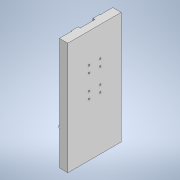
# Autodesk Inventor part: Zplita
Saved by Autodesk Inventor 2020.1 (Build 241239000, 239)
## iProperties
Created: 2023-01-09
Part Number: Zplita
Material: Типовые
Document SubType Name: Modeling
Designer: KirikDK
Density: 1 g/cm^3
Appearance: По умолчанию
Author: KirikDK
Autodesk Inventor part; units mm, degrees
ref_plane "YZ Plane" through (0, 0, 0) normal (1, 0, 0) x (0, 1, 0)
ref_plane "XZ Plane" through (0, 0, 0) normal (0, 1, 0) x (-1, 0, 0)
ref_plane "XY Plane" through (0, 0, 0) normal (0, 0, 1) x (1, 0, 0)
sketch "Эскиз1" plane through (0, 0, 0) normal (0, 1, 0) x (-1, 0, 0)
  line L0 (0, 94.5239) -> (-30, 94.5239)
  line L1 (-30, 94.5239) -> (-30, -95.4761)
  line L2 (-30, -95.4761) -> (0, -95.4761)
  line L3 (0, -95.4761) -> (0, 94.5239)
  line L4 (-30, 50.5239) -> (2, 50.5239)
  line L5 (2, 50.5239) -> (2, -51.4761)
  line L6 (2, -51.4761) -> (-30, -51.4761)
  line L7 (-30, -51.4761) -> (-30, 50.5239)
  point P0 (0, 0)
  point P1 (0, -51.4761)
  point P2 (0, 50.5239)
  dimension "d0" = 190
  dimension "d2" = 30
  dimension "d3" = 32
  dimension "d4" = 44
  dimension "d13" = 44
  constraints: 16 end point, 4 parallel, 2 horizontal, 2 perpendicular, 1 point on line
  measures "d0" distance of L2.end L0.start
  measures "d2" distance of L0.start L0.end
  measures "d3" distance of L4.start L4.end
  measures "d4" distance between parallel lines of L0 L4
  measures "d13" distance between parallel lines of L6 L2
extrude "Выдавливание1" add sketch "Эскиз1" along normal blind 400
sketch "Эскиз2" plane through (-2, 0, -51.4761) normal (-1, 0, 0) x (0, 0, 1)
  line L0 (25, -29) -> (77, -29)
  line L1 (77, -29) -> (77, 456)
  line L2 (77, 456) -> (25, 456)
  line L3 (25, 456) -> (25, -29)
  line L4 (0, 0) -> (102, 0) projected
  line L5 (102, 0) -> (102, 400) projected
  line L6 (0, 400) -> (102, 400) projected
  line L7 (0, 0) -> (0, 400) projected
  point P0 (51.4761, 0)
  point P1 (77, 400)
  point P2 (25, 400)
  point P3 (25, 0)
  point P4 (77, 0)
  dimension "d8" = 25
  dimension "d9" = 25
  dimension "d10" = 52
  constraints: 8 end point, 2 parallel, 1 horizontal, 1 perpendicular
  measures "d8" distance between parallel lines of L7 L3
  measures "d9" distance between parallel lines of L5 L1
  measures "d10" distance of L0.start L0.end
extrude "Выдавливание2" cut sketch "Эскиз2" against normal blind 7.4 contours L3 L6 L1 L4
sketch "Эскиз3" plane through (-2, 0, 50.5239) normal (-1, 0, 0) x (0, 0, 1)
  line L0 (44, 0) -> (44, 400) projected
  line L1 (-146, 0) -> (-146, 400) projected
  line L2 (44, 130.4195) -> (-146, 130.4195)
  line L3 (-146, 130.4195) -> (-146, 122.295)
  line L4 (-146, 122.295) -> (44, 122.295)
  line L5 (44, 122.295) -> (44, 130.4195)
  line L6 (-25, 400) -> (-25, 0) projected
  line L7 (-25, 0) -> (0, 0) projected
  line L8 (0, 0) -> (0, 400) projected
  line L9 (-25, 400) -> (0, 400) projected
  line L10 (-77, 0) -> (-77, 400) projected
  line L11 (-102, 400) -> (-77, 400) projected
  line L12 (-102, 0) -> (-102, 400) projected
  line L13 (-102, 0) -> (-77, 0) projected
  point P0 (-50.5239, 0)
  point P1 (0, 130.4195)
  point P2 (0, 122.295)
  point P3 (-102, 122.295)
  point P4 (-102, 130.4195)
  constraints: 8 end point, 2 parallel, 2 point on line, 1 horizontal, 1 perpendicular
extrude "Выдавливание3" add sketch "Эскиз3" against normal blind 10 contours L4 L8 L2 L0 | L4 L1 L2 L12
sketch "Эскиз4" plane through (5.4, 0, -51.4761) normal (-1, 0, 0) x (0, 0, 1)
  line L0 (76.5, 183) -> (25.5, 183)
  line L1 (76.5, 222) -> (76.5, 183)
  line L2 (25.5, 222) -> (76.5, 222)
  line L3 (25.5, 183) -> (25.5, 222)
  circle A0 centre (71, 190.5) radius 2.75
  circle A1 centre (31, 190.5) radius 2.75
  circle A2 centre (31, 214.5) radius 2.75
  circle A3 centre (71, 214.5) radius 2.75
  line L4 (76, 263) -> (77, 263)
  line L5 (76.5, 263) -> (76.5, 222)
  line L6 (76.5, 263) -> (25.5, 263)
  line L7 (76.5, 302) -> (76.5, 263)
  line L8 (25.5, 302) -> (76.5, 302)
  line L9 (25.5, 263) -> (25.5, 302)
  circle A4 centre (71, 270.5) radius 2.75
  circle A5 centre (31, 270.5) radius 2.75
  circle A6 centre (31, 294.5) radius 2.75
  circle A7 centre (71, 294.5) radius 2.75
  point P0 (51.4761, 0)
  point P1 (51, 182.5)
  point P2 (51, 262.5)
  constraints: 20 end point, 8 centre point, 1 horizontal, 1 vertical
extrude "Выдавливание4" cut sketch "Эскиз4" against normal blind 33 contours A0 | A1 | A2 | A3 | A4 | A5 | A6 | A7
